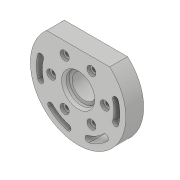
# Autodesk Inventor part: Ch5_tut1
Saved by Autodesk Inventor 2017 (Build 210142000, 142)
## iProperties
Created: 2016-07-11
Part Number: Ch5_tut1
Material: Generic
Document SubType Name: Modeling
Designer: anand
Density: 1 g/cm^3
Appearance: Default
Author: anand
Autodesk Inventor part; units mm, degrees
ref_plane "YZ Plane" through (0, 0, 0) normal (1, 0, 0) x (0, 1, 0)
ref_plane "XZ Plane" through (0, 0, 0) normal (0, 1, 0) x (-1, 0, 0)
ref_plane "XY Plane" through (0, 0, 0) normal (0, 0, 1) x (1, 0, 0)
sketch "Sketch1" plane through (0, 0, 0) normal (0, 0, 1) x (1, 0, 0)
  arc A0 (-10.5987, 11.9888) -> (10.5987, 11.9888) centre (0, 0) ccw
  line L0 (-10.5987, 11.9888) -> (10.5987, 11.9888)
  arc A1 (12.5617, -3.3659) -> (12.5617, 3.3659) centre (0, 0) ccw construction
  arc A2 (13.5185, -3.6223) -> (13.5185, 3.6223) centre (0, 0) ccw
  arc A3 (11.6048, -3.1095) -> (11.6048, 3.1095) centre (0, 0) ccw
  arc A4 (11.6048, -3.1095) -> (13.5185, -3.6223) centre (12.5617, -3.3659) ccw
  arc A5 (13.5185, 3.6223) -> (11.6048, 3.1095) centre (12.5617, 3.3659) ccw
  line L1 (0, 0) -> (20.2969, 0) construction
  arc A6 (3.6223, -13.5185) -> (9.8962, -9.8962) centre (0, 0) ccw
  arc A7 (3.1095, -11.6048) -> (3.6223, -13.5185) centre (3.3659, -12.5617) ccw
  arc A8 (3.1095, -11.6048) -> (8.4953, -8.4953) centre (0, 0) ccw
  arc A9 (9.8962, -9.8962) -> (8.4953, -8.4953) centre (9.1958, -9.1958) ccw
  arc A10 (3.3659, -12.5617) -> (9.1958, -9.1958) centre (0, 0) ccw construction
  arc A11 (-9.8962, -9.8962) -> (-3.6223, -13.5185) centre (0, 0) ccw
  arc A12 (-8.4953, -8.4953) -> (-9.8962, -9.8962) centre (-9.1958, -9.1958) ccw
  arc A13 (-8.4953, -8.4953) -> (-3.1095, -11.6048) centre (0, 0) ccw
  arc A14 (-3.6223, -13.5185) -> (-3.1095, -11.6048) centre (-3.3659, -12.5617) ccw
  arc A15 (-9.1958, -9.1958) -> (-3.3659, -12.5617) centre (0, 0) ccw construction
  arc A16 (-13.5185, 3.6223) -> (-13.5185, -3.6223) centre (0, 0) ccw
  arc A17 (-11.6048, 3.1095) -> (-13.5185, 3.6223) centre (-12.5617, 3.3659) ccw
  arc A18 (-11.6048, 3.1095) -> (-11.6048, -3.1095) centre (0, 0) ccw
  arc A19 (-13.5185, -3.6223) -> (-11.6048, -3.1095) centre (-12.5617, -3.3659) ccw
  arc A20 (-12.5617, 3.3659) -> (-12.5617, -3.3659) centre (0, 0) ccw construction
  dimension "d0" = 27.9908
  dimension "d1" = 16.002
  dimension "d2" = 30
  dimension "d3" = 13.0048
  dimension "d4" = 0.9906
  dimension "d7" = 180
  constraints: 42 point on circle, 21 centre point, 4 end point, 4 tangent, 2 coincident, 2 horizontal, 38 other
  measures "d1" radius of A0
  measures "d3" radius of A1
  measures "d4" radius of A4
extrude "Extrusion1" add sketch "Sketch1" along normal blind 5.9944
sketch "Sketch2" plane through (0, 0, 0) normal (0, 0, -1) x (-1, 0, 0)
  circle A0 centre (0, 0) radius 5.9944
  dimension "d11" = 11.9888
  constraints: 1 centre point, 1 coincident
  measures "d11" diameter of A0
extrude "Extrusion2" add sketch "Sketch2" along normal blind 1.9812
hole "Hole1" at (0, 0, 5.9944) direction (0, 0, -1) diameter 8.001 end through all counterbore diameter 9.9822 counterbore depth 1.9812
sketch "Sketch3" plane through (0, 0, 5.9944) normal (0, 0, 1) x (1, 0, 0)
  point P0 (0, 0)
  point P1 (8.9916, 0)
  dimension "d23" = 8.9916
  constraints: 1 horizontal alignment
  measures "d23" distance of point (0, 0) point (8.992, 0)
hole "Hole2" at (8.9916, 0, 5.9944) direction (0, 0, -1) diameter 1.4224 depth 5.6896 tip angle 118 counterbore diameter 2.9972 counterbore depth 0.9906
pattern_circular "Circular Pattern1" count 6 over 360 about axis through (0, 0, 0) along (0, 0, 1) of "Hole2"
chamfer "Chamfer1" distance 0.9906 angle 30 1 edges at (0, 4.9911, 5.9944) measured on face at (0.4016, -4.9749, 5.334)
body "Solid1"
